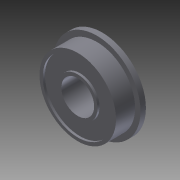
# Autodesk Inventor part: .375 ID .875 OD bearing
Saved by Autodesk Inventor 2012 (Build 160160000, 160)
## iProperties
Created: 2012-08-08
Part Number: .375 ID .875 OD bearing
Material: Default
Document SubType Name: Modeling
Designer: Bryce
Density: 1 g/cm^3
Author: Bryce
Autodesk Inventor part; units mm, degrees
ref_plane "YZ Plane" through (0, 0, 0) normal (1, 0, 0) x (0, 1, 0)
ref_plane "XZ Plane" through (0, 0, 0) normal (0, 1, 0) x (-1, 0, 0)
ref_plane "XY Plane" through (0, 0, 0) normal (0, 0, 1) x (1, 0, 0)
sketch "Sketch1" plane through (0, 0, 0) normal (0, 0, 1) x (1, 0, 0)
  circle A0 centre (0, 0) radius 4.7625
  circle A1 centre (0, 0) radius 11.1125
  circle A2 centre (0, 0) radius 12.6873
  circle A3 centre (0, 0) radius 5.715
  circle A4 centre (0, 0) radius 10.16
  dimension "d0" = 9.525
  dimension "d1" = 22.225
  dimension "d2" = 25.3746
  dimension "d7" = 20.32
  dimension "d8" = 11.43
  constraints: 5 centre point, 5 coincident
  measures "d0" diameter of A0
  measures "d1" diameter of A1
  measures "d2" diameter of A2
  measures "d7" diameter of A4
  measures "d8" diameter of A3
extrude "Extrusion1" add sketch "Sketch1" along normal blind 7.112 contours A1 | A3 | A4
extrude "Extrusion2" add sketch "Sketch1" along normal blind 1.5748 contours A2
extrude "Extrusion3" cut sketch "Sketch1" along normal blind 0.635 contours A4
sketch "Sketch2" plane through (0, 0, 7.112) normal (0, 0, 1) x (1, 0, 0)
  circle A0 centre (0, 0) radius 5.715 projected
  circle A1 centre (0, 0) radius 10.16 projected
extrude "Extrusion4" cut sketch "Sketch2" against normal blind 0.635
body "Solid1"
